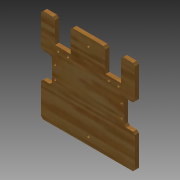
# Autodesk Inventor part: base
Saved by Autodesk Inventor 2013 (Build 170138000, 138)
## iProperties
Created: 2013-07-22
Part Number: base
Material: Generic
Document SubType Name: Modeling
Designer: pnyholm
Density: 1 g/cm^3
Author: pnyholm
Autodesk Inventor part; units mm, degrees
ref_plane "YZ Plane" through (0, 0, 0) normal (1, 0, 0) x (0, 1, 0)
ref_plane "XZ Plane" through (0, 0, 0) normal (0, 1, 0) x (-1, 0, 0)
ref_plane "XY Plane" through (0, 0, 0) normal (0, 0, 1) x (1, 0, 0)
sketch "Sketch1" plane through (0, 0, 0) normal (0, 0, 1) x (1, 0, 0)
  line L0 (0, 0) -> (152.4, 0)
  line L1 (152.4, 96.8375) -> (134.9375, 96.8375)
  line L2 (134.9375, 96.8375) -> (134.9375, 55.5625)
  line L3 (134.9375, 55.5625) -> (152.4, 55.5625)
  line L4 (0, 96.8375) -> (17.4625, 96.8375)
  line L5 (17.4625, 96.8375) -> (17.4625, 55.5625)
  line L6 (17.4625, 55.5625) -> (0, 55.5625)
  line L7 (152.4, 0) -> (152.4, 55.5625)
  line L8 (152.4, 96.8375) -> (152.4, 152.4)
  line L9 (0, 152.4) -> (0, 96.8375)
  line L10 (0, 55.5625) -> (0, 0)
  circle A0 centre (22.225, 86.6775) radius 2.1526
  circle A1 centre (22.225, 65.7225) radius 2.1526
  circle A2 centre (130.175, 86.6775) radius 2.1526
  circle A3 centre (130.175, 65.7225) radius 2.1526
  line L11 (22.479, 152.4) -> (22.479, 114.3)
  line L12 (22.479, 114.3) -> (47.879, 114.3)
  line L13 (47.879, 114.3) -> (47.879, 152.4)
  line L14 (104.521, 152.4) -> (104.521, 114.3)
  line L15 (104.521, 114.3) -> (129.921, 114.3)
  line L16 (129.921, 114.3) -> (129.921, 152.4)
  line L17 (22.479, 152.4) -> (0, 152.4)
  line L18 (152.4, 152.4) -> (129.921, 152.4)
  line L19 (104.521, 152.4) -> (47.879, 152.4)
  dimension "d0" = 152.4
  dimension "d1" = 152.4
  dimension "d2" = 41.275
  dimension "d3" = 55.5625
  dimension "d4" = 17.4625
  dimension "d5" = 41.275
  dimension "d6" = 17.4625
  dimension "d7" = 55.5625
  dimension "d8" = 152.4
  dimension "d10" = 4.3053
  dimension "d11" = 4.3053
  dimension "d12" = 4.3053
  dimension "d13" = 4.3053
  dimension "d15" = 22.225
  dimension "d16" = 22.225
  dimension "d17" = 22.225
  dimension "d18" = 22.225
  dimension "d19" = 10.16
  dimension "d20" = 10.16
  dimension "d21" = 10.16
  dimension "d22" = 10.16
  dimension "d28" = 107.442
  dimension "d29" = 25.4
  dimension "d30" = 25.4
  dimension "d31" = 22.479
  dimension "d32" = 38.1
  constraints: 40 end point, 18 perpendicular, 10 parallel, 4 centre point, 4 collinear, 1 horizontal
  measures "d0" distance of L9.start L8.end
  measures "d1" distance of L0.end L8.end
  measures "d2" distance of L1.end L2.end
  measures "d3" distance between parallel lines of L0 L3
  measures "d4" distance of L2.end L3.end
  measures "d5" distance of L4.end L5.end
  measures "d6" distance of L5.end L6.end
  measures "d7" distance between parallel lines of L0 L6
  measures "d8" distance between parallel lines of L10 L7
  measures "d10" diameter of A0
  measures "d11" diameter of A1
  measures "d12" diameter of A2
  measures "d13" diameter of A3
  measures "d15" distance from line of L9 A0.centre
  measures "d16" distance from line of L10 A1.centre
  measures "d17" distance from line of L8 A2.centre
  measures "d18" distance from line of L7 A3.centre
  measures "d19" distance from line of L4 A0.centre
  measures "d20" distance from line of L6 A1.centre
  measures "d21" distance from line of L1 A2.centre
  measures "d22" distance from line of L3 A3.centre
  measures "d28" distance between parallel lines of L16 L11
  measures "d29" distance of L11.end L12.end
  measures "d30" distance of L14.end L15.end
  measures "d31" distance between parallel lines of L16 L8
  measures "d32" distance of L12.end L13.end
extrude "Extrusion1" add sketch "Sketch1" along normal blind 6.35
chamfer "Chamfer1" distance 3.175 angle 45 12 edges at (0, 55.5625, 3.175) (17.4625, 55.5625, 3.175) (17.4625, 96.8375, 3.175) (0, 96.8375, 3.175) (152.4, 55.5625, 3.175) (134.9375, 55.5625, 3.175) (134.9375, 96.8375, 3.175) (152.4, 96.8375, 3.175) (152.4, 0, 3.175) (0, 0, 3.175) (0, 152.4, 3.175) (152.4, 152.4, 3.175)
chamfer "Chamfer2" distance 3.175 angle 45 4 edges at (22.479, 152.4, 3.175) (47.879, 152.4, 3.175) (104.521, 152.4, 3.175) (129.921, 152.4, 3.175)
sketch "Sketch2" plane through (0, 0, 0) normal (0, 0, -1) x (-1, 0, 0)
  line L0 (-22.479, 114.3) -> (-22.479, 149.225) projected
  line L1 (-129.921, 114.3) -> (-104.521, 114.3) projected
  line L2 (-129.921, 149.225) -> (-129.921, 114.3) projected
  line L3 (-125.1585, 107.95) -> (-27.2415, 107.95) construction
  point P0 (0, 0)
  point P1 (-109.2835, 107.95)
  point P2 (-43.1165, 107.95)
  dimension "d37" = 15.875
  dimension "d39" = 15.875
  dimension "d40" = 4.7625
  dimension "d41" = 4.7625
  dimension "d42" = 6.35
  constraints: 2 end point, 2 point on line, 1 coincident, 1 horizontal, 1 perpendicular
  measures "d37" distance of point (-109.283, 107.95) point (-125.158, 107.95)
  measures "d39" distance of L3.end point (-43.116, 107.95)
  measures "d40" distance from line of L0 L3.end
  measures "d41" distance from line of point (-125.158, 107.95) L2
  measures "d42" distance between parallel lines of L3 L1
hole "Hole1" at (109.2835, 107.95, 0) at (43.1165, 107.95, 0) at (27.2415, 107.95, 0) at (125.1585, 107.95, 0) direction (0, 0, 1) diameter 4.3053 end through all
sketch "Sketch3" plane through (0, 0, 6.35) normal (0, 0, 1) x (1, 0, 0)
  line L0 (101.346, 152.4) -> (51.054, 152.4) projected
  line L1 (3.175, 0) -> (149.225, 0) projected
  point P0 (0, 0)
  point P1 (76.2, 139.7)
  point P2 (76.2, 12.7)
  dimension "d50" = 76.2
  dimension "d51" = 76.2
  dimension "d52" = 12.7
  dimension "d53" = 12.7
  measures "d50" horizontal distance of point (76.2, 12.7) point (0, 0)
  measures "d51" horizontal distance of point (0, 0) point (76.2, 139.7)
  measures "d52" distance from line of point (76.2, 139.7) L0
  measures "d53" distance from line of L1 point (76.2, 12.7)
hole "Hole2" at (76.2, 139.7, 6.35) at (76.2, 12.7, 6.35) direction (0, 0, -1) diameter 4.4958 end through all
equation "\"d31\" = -0.5 * d28 + 0.5 * d0"
equation "\"d41\" = d40"
body "Solid1"
